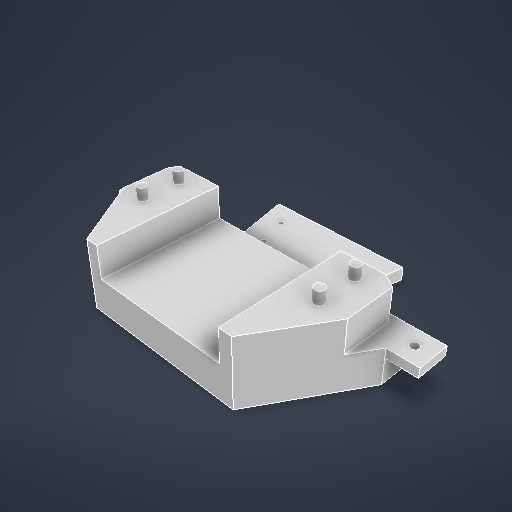
# Autodesk Inventor part: Front Bridge
Saved by Autodesk Inventor 2025 (Build 290162000, 162)
## iProperties
Created: 2024-05-23
Part Number: Front Bridge
Material: Generic
Document SubType Name: Modeling
Designer: DELL
Density: 1 g/cm^3
Appearance: Default
Mass: 43.2187 g
Surface Area: 102.411 cm^2
Volume: 43.2187 cm^3
Author: DELL
Autodesk Inventor part; units mm, degrees
ref_plane "YZ Plane" through (0, 0, 0) normal (1, 0, 0) x (0, 1, 0)
ref_plane "XZ Plane" through (0, 0, 0) normal (0, 1, 0) x (-1, 0, 0)
ref_plane "XY Plane" through (0, 0, 0) normal (0, 0, 1) x (1, 0, 0)
derived "Car_Plan.ipt"
sketch "Car_Sketch" plane through (0, 0, 0) normal (0, 1, 0) x (-1, 0, 0)
  line L0 (0, 0) -> (94, 0)
  line L1 (0, 0) -> (0, 105)
  line L2 (94, 0) -> (94, 105)
  line L3 (0, 105) -> (20, 105)
  line L4 (20, 105) -> (20, 190)
  line L5 (20, 190) -> (74, 190)
  line L6 (74, 190) -> (74, 105)
  line L7 (74, 105) -> (94, 105)
  line L8 (-5, 68) -> (-5, 0)
  line L9 (-5, 0) -> (-32, 0)
  line L10 (-32, 0) -> (-32, 68)
  line L11 (-32, 68) -> (-5, 68)
  line L12 (47, 190) -> (47, 0) construction
  line L13 (126, 68) -> (99, 68)
  line L14 (99, 68) -> (99, 0)
  line L15 (126, 0) -> (126, 68)
  line L16 (99, 0) -> (126, 0)
  line L17 (-5, 34) -> (99, 34) construction
  line L18 (0, 95) -> (94, 95) construction
  line L19 (-5, 190) -> (-32, 190)
  line L20 (-32, 122) -> (-5, 122)
  line L21 (-32, 190) -> (-32, 122)
  line L22 (-5, 122) -> (-5, 190)
  line L23 (-5, 156) -> (99, 156) construction
  line L24 (126, 122) -> (99, 122)
  line L25 (126, 190) -> (126, 122)
  line L26 (99, 190) -> (126, 190)
  line L27 (99, 122) -> (99, 190)
  line L28 (0, 156) -> (47, 34) construction
  line L29 (94, 156) -> (47, 34) construction
  line L30 (0, 156) -> (-174.2341, 34) construction
  line L31 (-5, 34) -> (-174.2341, 34) construction
  line L32 (8.9873, 132.6713) -> (47, 141.55) construction
  line L33 (85.0127, 132.6713) -> (47, 141.55) construction
sketch "Front_Bridge_Base" plane through (0, 0, 0) normal (0, 1, 0) x (-1, 0, 0)
  circle A0 centre (0, 156) radius 1
  circle A1 centre (94, 156) radius 1
  line L0 (-5, 161) -> (-5, 151)
  line L1 (-5, 151) -> (29.5, 151)
  line L2 (99, 151) -> (99, 161)
  line L3 (99, 161) -> (90, 161)
  line L4 (4, 161) -> (22, 190)
  line L5 (22, 190) -> (72, 190)
  line L6 (72, 190) -> (90, 161)
  line L7 (0, 156) -> (94, 156) construction
  line L8 (4, 161) -> (-5, 161)
  line L9 (40.95, 172.3) -> (53.05, 172.3)
  line L10 (53.05, 172.3) -> (53.05, 149.9)
  line L11 (53.05, 149.9) -> (40.95, 149.9)
  line L12 (40.95, 149.9) -> (40.95, 172.3)
  line L13 (47, 156) -> (47, 149.9) construction
  line L14 (32, 151) -> (37, 144)
  line L15 (37, 144) -> (57, 144)
  line L16 (57, 144) -> (62, 151)
  line L17 (47, 156) -> (47, 144) construction
  line L18 (32, 151) -> (62, 151)
  line L19 (62, 151) -> (64.5, 151)
  line L20 (29.5, 151) -> (24.5, 126)
  line L21 (24.5, 126) -> (69.5, 126)
  line L22 (69.5, 126) -> (64.5, 151)
  line L23 (64.5, 151) -> (99, 151)
  line L24 (29.5, 151) -> (32, 151)
  line L25 (4, 161) -> (4, 151)
  line L26 (90, 161) -> (90, 151)
  circle A2 centre (32, 133) radius 1
  circle A3 centre (35, 143) radius 1
  line L27 (47, 156) -> (47, 126) construction
  circle A4 centre (62, 133) radius 1
  circle A5 centre (59, 143) radius 1
  line L28 (9, 169.0556) -> (9, 151)
  line L29 (84.8333, 151) -> (84.5992, 150.8961)
  line L30 (85, 169.0556) -> (85, 151)
  line L31 (26, 190) -> (26, 151)
  line L32 (68, 190) -> (68, 151)
  circle A6 centre (17, 157) radius 1.5
  circle A7 centre (17, 169) radius 1.5
  circle A8 centre (77, 157) radius 1.5
  circle A9 centre (77, 169) radius 1.5
  dimension "d130" = 2
  dimension "d131" = 2
  dimension "d132" = 5
  dimension "d134" = 5
  dimension "d136" = 5
  dimension "d137" = 5
  dimension "d138" = 4
  dimension "d139" = 5
  dimension "d140" = 34
  dimension "d143" = 50
  dimension "d168" = 16.3
  dimension "d169" = 12.1
  dimension "d170" = 22.4
  dimension "d173" = 6.05
  dimension "d174" = 12
  dimension "d175" = 20
  dimension "d176" = 15
  dimension "d214" = 45
  dimension "d215" = 30
  dimension "d216" = 35
  dimension "d221" = 2
  dimension "d222" = 2
  dimension "d223" = 8
  dimension "d224" = 18
  dimension "d225" = 12
  dimension "d226" = 15
  dimension "d252" = 5
  dimension "d253" = 5
  dimension "d254" = 4
  dimension "d255" = 4
  dimension "d277" = 3
  dimension "d281" = 3
  dimension "d282" = 3
  dimension "d283" = 3
  dimension "d284" = 8
  dimension "d285" = 8
  dimension "d286" = 8
  dimension "d287" = 8
  dimension "d288" = 6
  dimension "d289" = 18
  dimension "d290" = 6
  dimension "d291" = 18
  constraints: 66 end point, 21 perpendicular, 12 point on line, 11 parallel, 10 centre point, 5 equal length, 4 midpoint, 2 coincident, 2 symmetric about line, 2 other
  measures "d130" diameter of A0
  measures "d131" diameter of A1
  measures "d132" distance from line of L0 L7.start
  measures "d134" distance from line of L1 point (0, 156)
  measures "d136" distance from line of L2 point (94, 156)
  measures "d137" distance from line of L3 point (94, 156)
  measures "d138" horizontal distance of L4.start point (0, 156)
  measures "d139" distance from line of L8 L7.start
  measures "d140" distance between parallel lines of L7 L5
  measures "d143" distance of L4.end L5.end
  measures "d168" distance from line of L9 L13.start
  measures "d169" distance of L10.end L11.end
  measures "d170" distance of L10.end L9.end
  measures "d173" distance between parallel lines of L12 L13
  measures "d174" distance of L17.end L13.start
  measures "d175" distance of L15.end L14.end
  measures "d176" distance from line of L17 L14.start
  measures "d214" distance of L20.end L21.end
  measures "d215" distance between parallel lines of L21 L7
  measures "d216" distance of L1.end L19.end
  measures "d221" diameter of A2
  measures "d222" diameter of A3
  measures "d223" distance from line of A3.centre L18
  measures "d224" distance from line of A2.centre L24
  measures "d225" distance from line of L27 A3.centre
  measures "d226" distance from line of L27 A2.centre
  measures "d252" distance between parallel lines of L28 L25
  measures "d253" distance between parallel lines of L26 L30
  measures "d254" distance from line of L4.end L31
  measures "d255" distance from line of L32 L5.end
  measures "d277" diameter of A6
  measures "d281" diameter of A7
  measures "d282" diameter of A8
  measures "d283" diameter of A9
  measures "d284" distance from line of L28 A6.centre
  measures "d285" distance from line of A7.centre L28
  measures "d286" distance from line of L30 A8.centre
  measures "d287" distance from line of L30 A9.centre
  measures "d288" distance from line of L1 A6.centre
  measures "d289" distance from line of L1 A7.centre
  measures "d290" distance from line of L23 A8.centre
  measures "d291" distance from line of L23 A9.centre
extrude "Base_1_Extrusion" add sketch "Front_Bridge_Base" along normal blind 3 contours L8 L25 L1 L0 | L4 L28 L1 L25 | L4 L5 L31 L1 L28 | L31 L5 L32 L23 L19 L18 L10 L9 L12 L24 L1 | L5 L6 L30 L23 L32 | L12 L9 L10 L18 | L6 L26 L23 L30 | L3 L2 L23 L26 | A6 | A7 | A8 | A9
sketch "Base_2" plane through (0, 3, 0) normal (0, 1, 0) x (1, 0, 0)
  line L0 (-9, -169.0556) -> (-9, -151) projected
  line L1 (-4, -161) -> (-22, -190) projected
  line L2 (5, -151) -> (-29.5, -151) projected
  line L3 (-26, -190) -> (-26, -151) projected
  line L4 (-22, -190) -> (-72, -190) projected
  line L5 (-68, -190) -> (-68, -151) projected
  line L6 (-72, -190) -> (-90, -161) projected
  line L7 (-85, -169.0556) -> (-85, -151) projected
  line L8 (-64.5, -151) -> (-99, -151) projected
  point P0 (0, 0)
extrude "Base_2_Extrusion" add sketch "Base_2" along normal blind 10
extrude "Bottom_Base_Extrusion" add sketch "Front_Bridge_Base" against normal blind 8 contours L4 L28 L1 L25 | L4 L5 L31 L1 L28 | L31 L5 L32 L23 L19 L18 L10 L9 L12 L24 L1 | L5 L6 L30 L23 L32 | L12 L9 L10 L18 | L6 L26 L23 L30 | A6 | A7 | A8 | A9
chamfer "Chamfer_For_Wheel_Anchor" distance 4 angle 33 2 edges at (-9, 8, 151) (-85, 8, 151) measured on face at (-9.5, 8, 151) measured on face at (-84.5, 8, 151)
sketch "Chassis_Connector" plane through (0, -8, 0) normal (0, -1, 0) x (1, 0, 0)
  line L0 (-29.5, 151) -> (-24.5, 126) projected
  line L1 (-24.5, 126) -> (-69.5, 126) projected
  line L2 (-69.5, 126) -> (-64.5, 151) projected
  line L3 (-29.5, 151) -> (-32, 151) projected
  line L4 (-32, 151) -> (-62, 151) projected
  line L5 (-62, 151) -> (-64.5, 151) projected
  circle A0 centre (-35, 143) radius 1 projected
  circle A1 centre (-32, 133) radius 1 projected
  circle A2 centre (-62, 133) radius 1 projected
  circle A3 centre (-59, 143) radius 1 projected
  point P0 (0, 0)
extrude "Chassis_Connector_Extrusion" add sketch "Chassis_Connector" against normal blind 4
sketch "Alignment_Pin" plane through (0, 13, 0) normal (0, 1, 0) x (1, 0, 0)
  circle A0 centre (-17, -157) radius 1.5 projected
  circle A1 centre (-17, -169) radius 1.5 projected
  circle A2 centre (-77, -169) radius 1.5 projected
  circle A3 centre (-77, -157) radius 1.5 projected
  point P0 (0, 0)
extrude "Alignment_Pin_Extrusion" add sketch "Alignment_Pin" along normal blind 4
thicken "Thicken1" operation cut thickness 0.3 both sides no extend neighbours no toward (-0.8451901, 0, -0.5344658) faces at (-0.8452, 2, 155.4655)
thicken "Thicken2" operation cut thickness 0.3 both sides no extend neighbours no toward (-0.6324454, 0, 0.774605) faces at (-94.6324, 2, 156.7746)
body "Solid3"
